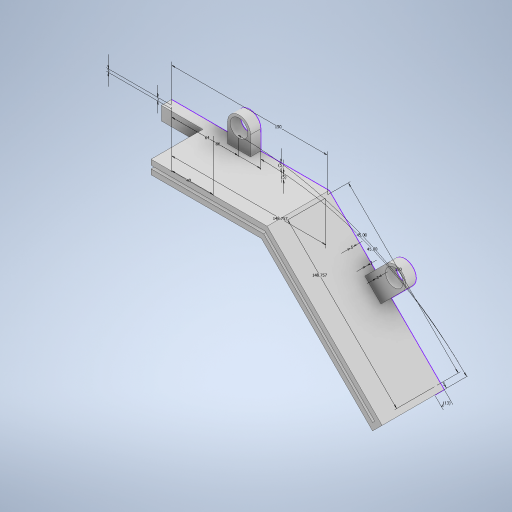
# Autodesk Inventor part: hold_right
Saved by Autodesk Inventor 2024 (Build 280153000, 153)
## iProperties
Created: 2024-02-27
Part Number: hold_right
Material: Generic
Document SubType Name: Modeling
Designer: Administrator
Density: 1 g/cm^3
Appearance: Default
Author: Administrator
Autodesk Inventor part; units mm, degrees
ref_plane "YZ Plane" through (0, 0, 0) normal (1, 0, 0) x (0, 1, 0)
ref_plane "XZ Plane" through (0, 0, 0) normal (0, 1, 0) x (-1, 0, 0)
ref_plane "XY Plane" through (0, 0, 0) normal (0, 0, 1) x (1, 0, 0)
sketch "Sketch1" plane through (0, 0, 0) normal (0, 0, 1) x (1, 0, 0)
  line L0 (-127.5811, 34.9091) -> (-127.5811, 31.9091)
  line L1 (-127.5811, 34.9091) -> (-127.5811, 39.9091)
  line L2 (-127.5811, 31.9091) -> (-127.5811, 26.9091)
  line L3 (-127.5811, 26.9091) -> (19.1052, 26.9091)
  line L4 (-127.5811, 31.9091) -> (21.1763, 31.9091)
  line L5 (22.4189, 34.9091) -> (-127.5811, 34.9091)
  line L6 (24.49, 39.9091) -> (-127.5811, 39.9091)
  line L7 (126.3636, -73.2783) -> (21.1763, 31.9091)
  line L8 (22.4189, 34.9091) -> (128.4849, -71.157)
  line L9 (128.4849, -71.157) -> (126.3636, -73.2783)
  line L10 (19.1052, 26.9091) -> (126.3636, -80.3493)
  line L11 (135.556, -71.157) -> (24.49, 39.9091)
  line L12 (126.3636, -80.3493) -> (135.556, -71.157)
  line L13 (-87.5811, 26.9091) -> (-87.5811, 31.9091)
  line L14 (105.1971, 0.6309) -> (84.4826, -20.0836)
  circle A0 centre (97.4189, 8.4091) radius 8.5
  circle A1 centre (97.4189, 8.4091) radius 11
  line L15 (89.6407, 16.1872) -> (68.9263, -4.5272)
  line L16 (55.1971, -49.3691) -> (75.2902, -29.276)
  line L17 (39.6407, -33.8128) -> (59.7339, -13.7196)
  circle A2 centre (47.4189, -41.5909) radius 8.5
  circle A3 centre (47.4189, -41.5909) radius 11
  line L18 (-41.5811, 8.4091) -> (-41.5811, 26.9091)
  line L19 (-63.5811, 8.4091) -> (-63.5811, 26.9091)
  circle A4 centre (-52.5811, 8.4091) radius 8.5
  circle A5 centre (-52.5811, 8.4091) radius 11
  line L20 (-41.5811, 58.4091) -> (-41.5811, 39.9091)
  circle A6 centre (-52.5811, 58.4091) radius 8.5
  circle A7 centre (-52.5811, 58.4091) radius 11
  line L21 (-63.5811, 58.4091) -> (-63.5811, 39.9091)
  line L22 (-87.5811, 34.9091) -> (-87.5811, 39.9091)
  point P0 (0, 0)
  point P1 (-127.5811, 33.4091)
  point P2 (-127.5811, 33.4091)
  point P3 (-127.5811, 29.4091)
  point P4 (-87.5811, 29.4091)
  point P5 (-51.5456, 39.9091)
  dimension "d0" = 3
  dimension "d1" = 3
  dimension "d2" = 5
  dimension "d3" = 5
  dimension "d4" = 5
  dimension "d5" = 3
  dimension "d6" = 5
  dimension "d7" = 150
  dimension "d8" = 148.7574
  dimension "d9" = 148.7574
  dimension "d10" = 150
  dimension "d11" = 13
  dimension "d12" = 5
  dimension "d13" = 40
  dimension "d14" = 45
  dimension "d15" = 45
  dimension "d16" = 86
  dimension "d17" = 64
  constraints: 46 end point, 8 centre point, 8 point on circle, 5 point on line, 4 coincident, 3 midpoint, 2 perpendicular, 1 parallel, 1 tangent
  measures "d0" distance of L0.start L0.end
  measures "d1" distance between parallel lines of L4 L5
  measures "d2" distance between parallel lines of L5 L6
  measures "d3" distance between parallel lines of L3 L4
  measures "d4" distance between parallel lines of L7 L10
  measures "d5" distance between parallel lines of L8 L7
  measures "d6" distance between parallel lines of L11 L8
  measures "d7" distance of L8.start L0.start
  measures "d8" distance of L0.end L7.end
  measures "d9" distance of L7.start L7.end
  measures "d10" distance of L8.start L8.end
  measures "d11" distance of L10.end L11.start
  measures "d12" distance between parallel lines of L9 L12
  measures "d13" distance of point (-127.581, 29.409) point (-87.581, 29.409)
  measures "d14" angle of L20 L12
  measures "d15" angle of L21 L12
  measures "d16" distance from line of point (-127.581, 33.409) L20
  measures "d17" distance from line of point (-127.581, 33.409) L21
extrude "Extrusion1" add sketch "Sketch1" along normal blind 10 contours L5 L8 L9 L7 L4 L0 | L4 L13 L3 L2 | L21 A7 L20 L6 | L3 L18 A5 L19 | A7 | A5 | L15 A1 L14 L11 | L10 L16 A3 L17 | A1 | A3
extrude "Extrusion2" add sketch "Sketch1" along normal blind 60 contours L1 L6 L22 L5 | L22 L6 L11 L12 L10 L3 L13 L4 L7 L9 L8 L5
sketch "Sketch2" plane through (0, 0, 60) normal (0, 0, 1) x (1, 0, 0)
  line L0 (-127.5811, 39.9091) -> (-127.5811, 34.9091) projected
  line L1 (-127.5811, 34.9091) -> (22.4189, 34.9091) projected
  line L2 (-127.5811, 39.9091) -> (-87.5811, 39.9091)
  line L3 (-87.5811, 39.9091) -> (-87.5811, 34.9091)
  line L4 (-87.5811, 34.9091) -> (-127.5811, 34.9091)
  line L5 (-127.5811, 34.9091) -> (-127.5811, 39.9091)
  point P0 (0, 0)
  dimension "d22" = 40
  constraints: 8 end point, 2 parallel, 1 horizontal, 1 perpendicular, 1 point on line
  measures "d22" distance of L3.end L4.end
extrude "Extrusion3" cut sketch "Sketch2" against normal blind 50
body "Solid1"
